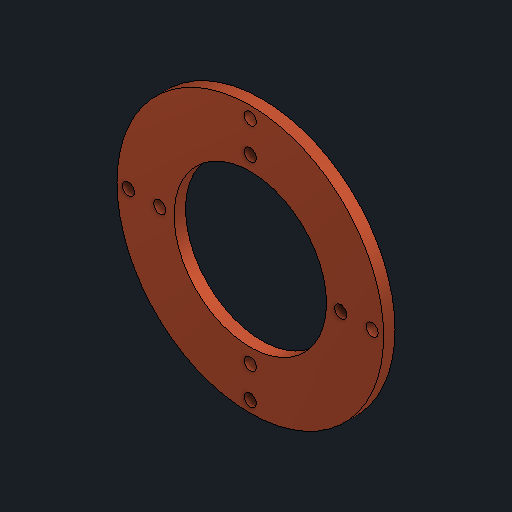
# Autodesk Inventor part: plasma_chamber_holder
Saved by Autodesk Inventor 2025 (Build 290162000, 162)
## iProperties
Created: 2024-05-15
Part Number: plasma_chamber_holder
Material: Copper
Document SubType Name: Modeling
Designer: kuzmin
Density: 8.94 g/cm^3
Appearance: Copper - Satin
Author: kuzmin
Autodesk Inventor part; units mm, degrees
ref_plane "YZ Plane" through (0, 0, 0) normal (1, 0, 0) x (0, 1, 0)
ref_plane "XZ Plane" through (0, 0, 0) normal (0, 1, 0) x (-1, 0, 0)
ref_plane "XY Plane" through (0, 0, 0) normal (0, 0, 1) x (1, 0, 0)
sketch "Sketch1" plane through (0, 0, 0) normal (0, 0, 1) x (1, 0, 0)
  circle A0 centre (0, 0) radius 20
  circle A1 centre (0, 0) radius 35
  dimension "d0" = 70
  dimension "d1" = 40
  constraints: 2 centre point, 2 coincident
  measures "d0" diameter of A1
  measures "d1" diameter of A0
extrude "Extrusion1" add sketch "Sketch1" along normal blind 3
sketch "Sketch2" plane through (0, 0, 3) normal (0, 0, 1) x (1, 0, 0)
  circle A0 centre (0, 0) radius 23.75 construction
  circle A1 centre (0, 0) radius 32 construction
  point P0 (23.75, 0)
  point P1 (32, 0)
  dimension "d4" = 64
  dimension "d5" = 47.5
  constraints: 4 horizontal alignment, 2 coincident, 4 other
hole "Hole1" at (23.75, 0, 3) at (32, 0, 3) direction (0, 0, -1) diameter 3.2 end through all
pattern_circular "Circular Pattern1" count 4 over 360 about axis through (0, 0, 0) along (0, 0, 1) of "Hole1"
body "Solid1"
